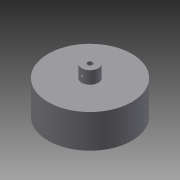
# Autodesk Inventor part: omni_wheel
Saved by Autodesk Inventor 2015 (Build 190159000, 159)
## iProperties
Created: 2017-09-27
Part Number: omni_wheel
Material: Generic
Document SubType Name: Modeling
Designer: Anshul
Density: 1 g/cm^3
Appearance: Default
Author: Anshul
Autodesk Inventor part; units mm, degrees
ref_plane "YZ Plane" through (0, 0, 0) normal (1, 0, 0) x (0, 1, 0)
ref_plane "XZ Plane" through (0, 0, 0) normal (0, 1, 0) x (-1, 0, 0)
sketch "Sketch1" plane through (0, 0, 0) normal (0, 1, 0) x (-1, 0, 0)
  circle A0 centre (0, 0) radius 50
  circle A1 centre (0, 0) radius 10
  circle A2 centre (0, 0) radius 3
  line L0 (10, 0) -> (-10, 0)
  dimension "d0" = 100
  dimension "d1" = 20
  dimension "d2" = 6
  constraints: 3 centre point, 3 coincident, 2 end point, 2 point on circle, 1 horizontal
  measures "d0" diameter of A0
  measures "d1" diameter of A1
  measures "d2" diameter of A2
extrude "Extrusion1" add sketch "Sketch1" against normal blind 40
extrude "Extrusion2" add sketch "Sketch1" along normal blind 15 contours L0 A2 A1 | A1 L0 A2
ref_plane "Work Plane1" through (-10, 0, 0) normal (0, 0, 1) x (1, 0, 0)
sketch "Sketch2" plane through (-10, 0, 0) normal (0, 0, 1) x (1, 0, 0)
  line L0 (20, 15) -> (0, 15) projected
  line L1 (10, 15) -> (10, 7.5)
  circle A0 centre (10, 7.5) radius 1.5
  point P0 (10, 0)
  dimension "d8" = 7.5
  dimension "d9" = 3
  constraints: 2 end point, 1 centre point, 1 coincident, 1 midpoint, 1 vertical
  measures "d8" distance of L1.start L1.end
  measures "d9" diameter of A0
extrude "Extrusion3" cut sketch "Sketch2" along normal mid plane 30
body "Solid1"
